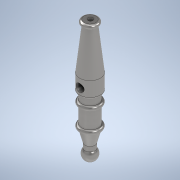
# Autodesk Inventor part: Cannon
Saved by Autodesk Inventor 2021 (Build 250183000, 183)
## iProperties
Created: 2021-02-06
Part Number: Cannon
Material: Iron, Malleable
Document SubType Name: Modeling
Designer: buntykrgdg
Density: 7.15 g/cm^3
Appearance: Semi-Polished
Author: buntykrgdg
Autodesk Inventor part; units mm, degrees
ref_plane "YZ Plane" through (0, 0, 0) normal (1, 0, 0) x (0, 1, 0)
ref_plane "XZ Plane" through (0, 0, 0) normal (0, 1, 0) x (-1, 0, 0)
ref_plane "XY Plane" through (0, 0, 0) normal (0, 0, 1) x (1, 0, 0)
sketch "Sketch1" plane through (0, 0, 0) normal (0, 1, 0) x (-1, 0, 0)
  arc A0 (8, 0) -> (-8, 0) centre (0, 0) ccw
  line L0 (8, 0) -> (-8, 0)
  point P0 (0, 0)
  dimension "d0" = 16
  dimension "d1" = 8
  constraints: 2 end point, 2 point on circle, 1 centre point, 1 horizontal
  measures "d0" distance of L0.start L0.end
  measures "d1" radius of A0
revolve "Revolution1" add sketch "Sketch1" angle 360 about axis through (-8, 0, 0) along (1, 0, 0)
sketch "Sketch2" plane through (0, 0, 0) normal (0, 1, 0) x (-1, 0, 0)
  circle A0 centre (0, 0) radius 6
  dimension "d3" = 12
  constraints: 1 centre point, 1 coincident
  measures "d3" diameter of A0
extrude "Extrusion1" add sketch "Sketch2" along normal blind 11
sketch "Sketch3" plane through (0, 0, 0) normal (0, 0, 1) x (1, 0, 0)
  line L0 (6, 11) -> (-6, 11) projected
  line L1 (0, 11) -> (0, 26)
  line L2 (0, 26) -> (10, 26)
  line L3 (10, 26) -> (6, 11)
  point P0 (0, 0)
  dimension "d6" = 15
  dimension "d7" = 10
  constraints: 6 end point, 1 midpoint, 1 perpendicular, 1 vertical
  measures "d6" distance of L1.start L1.end
  measures "d7" distance of L1.end L2.end
revolve "Revolution2" add sketch "Sketch3" angle 360 about axis through (0, 11, 0) along (0, 1, 0)
sketch "Sketch4" plane through (0, 0, 0) normal (0, 0, 1) x (1, 0, 0)
  line L0 (-10, 26) -> (10, 26) projected
  line L1 (0, 26) -> (0, 31)
  line L2 (0, 31) -> (-10, 31)
  arc A0 (-10, 31) -> (-10, 26) centre (-10, 28.5) ccw
  point P0 (0, 0)
  dimension "d9" = 5
  dimension "d10" = 10
  dimension "d11" = 2.5
  constraints: 4 end point, 2 point on circle, 1 centre point, 1 midpoint, 1 perpendicular, 1 vertical
  measures "d9" distance of L1.start L1.end
  measures "d10" distance of L1.end L2.end
  measures "d11" radius of A0
revolve "Revolution3" add sketch "Sketch4" angle 360 about axis through (0, 26, 0) along (0, 1, 0)
sketch "Sketch5" plane through (0, 31, 0) normal (0, 1, 0) x (1, 0, 0)
  point P0 (0, 0)
sketch "Sketch6" plane through (0, 31, 0) normal (0, 1, 0) x (1, 0, 0)
  circle A0 centre (0, 0) radius 10
  dimension "d13" = 20
  constraints: 1 centre point, 1 coincident
  measures "d13" diameter of A0
extrude "Extrusion2" add sketch "Sketch6" along normal blind 20
sketch "Sketch7" plane through (0, 0, 0) normal (0, 0, 1) x (1, 0, 0)
  line L0 (10, 51) -> (-10, 51) projected
  line L1 (0, 51) -> (0, 56)
  line L2 (0, 56) -> (-10, 56)
  arc A0 (-10, 56) -> (-10, 51) centre (-10, 53.5) ccw
  point P0 (0, 0)
  dimension "d16" = 5
  dimension "d17" = 10
  dimension "d18" = 2.5
  constraints: 4 end point, 2 point on circle, 1 centre point, 1 midpoint, 1 perpendicular, 1 vertical
  measures "d16" distance of L1.start L1.end
  measures "d17" distance of L1.end L2.end
  measures "d18" radius of A0
revolve "Revolution4" add sketch "Sketch7" angle 360 about axis through (0, 51, 0) along (0, 1, 0)
sketch "Sketch8" plane through (0, 56, 0) normal (0, 1, 0) x (1, 0, 0)
  circle A0 centre (0, 0) radius 10
  dimension "d20" = 20
  constraints: 1 centre point, 1 coincident
  measures "d20" diameter of A0
extrude "Extrusion3" add sketch "Sketch8" along normal blind 8
sketch "Sketch9" plane through (0, 64, 0) normal (0, 1, 0) x (1, 0, 0)
  circle A0 centre (0, 0) radius 12.5
  dimension "d23" = 25
  constraints: 1 centre point, 1 coincident
  measures "d23" diameter of A0
extrude "Extrusion4" add sketch "Sketch9" along normal blind 20
fillet "Fillet1" radius 2.5 1 edges at (-12.5, 64, 0)
sketch "Sketch10" plane through (0, 0, 0) normal (0, 0, 1) x (1, 0, 0)
  point P0 (0, 0)
sketch "Sketch11" plane through (0, 0, 0) normal (0, 0, 1) x (1, 0, 0)
  line L0 (12.5, 84) -> (-12.5, 84) projected
  line L1 (0, 84) -> (0, 134)
  line L2 (0, 134) -> (-7, 134)
  line L3 (-7, 134) -> (-12.5, 84)
  point P0 (0, 0)
  dimension "d27" = 50
  dimension "d28" = 7
  constraints: 6 end point, 1 midpoint, 1 perpendicular, 1 vertical
  measures "d27" distance of L1.start L1.end
  measures "d28" distance of L1.end L2.end
revolve "Revolution5" add sketch "Sketch11" angle 360 about axis through (0, 84, 0) along (0, 1, 0)
sketch "Sketch12" plane through (0, 0, 0) normal (0, 0, 1) x (1, 0, 0)
  line L0 (7, 134) -> (-7, 134) projected
  line L1 (0, 134) -> (0, 139)
  line L2 (0, 139) -> (-7, 139)
  arc A0 (-7, 139) -> (-7, 134) centre (-7, 136.5) ccw
  point P0 (0, 0)
  dimension "d30" = 5
  dimension "d31" = 7
  dimension "d32" = 2.5
  constraints: 4 end point, 2 point on circle, 1 centre point, 1 midpoint, 1 perpendicular, 1 vertical
  measures "d30" distance of L1.start L1.end
  measures "d31" distance of L1.end L2.end
  measures "d32" radius of A0
revolve "Revolution6" add sketch "Sketch12" angle 360 about axis through (0, 134, 0) along (0, 1, 0)
sketch "Sketch13" plane through (0, 0, 0) normal (0, 0, 1) x (1, 0, 0)
  circle A0 centre (0, 74) radius 4.7
  line L0 (7, 139) -> (-7, 139) projected
  point P0 (0, 0)
  dimension "d34" = 9.4
  dimension "d35" = 65
  constraints: 1 centre point
  measures "d34" diameter of A0
  measures "d35" distance from line of L0 A0.centre
extrude "Extrusion5" cut sketch "Sketch13" against normal through all both and the other way through all
sketch "Sketch14" plane through (0, 139, 0) normal (0, 1, 0) x (1, 0, 0)
  point P0 (0, 0)
  point P1 (0.1818, 0.4029)
hole "Hole1" at (0.1818, 139, -0.4029) direction (0, -1, 0) diameter 6 depth 50 tip angle 118
body "Solid1"
